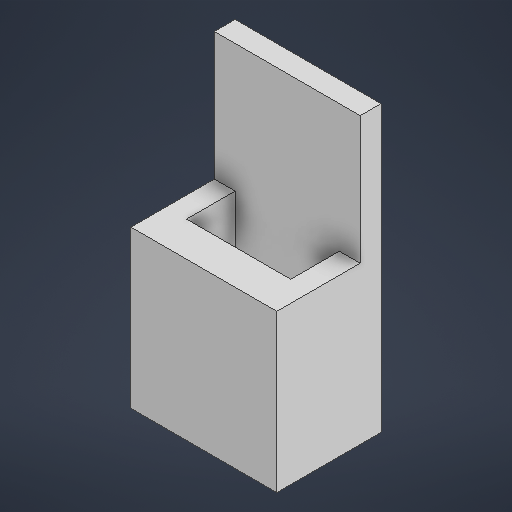
# Autodesk Inventor part: IRsensorhub
Saved by Autodesk Inventor 2026.2 (Build 302298000, 298)
## iProperties
Created: 2026-04-13
Part Number: IRsensorhub
Material: Generic
Document SubType Name: Modeling
Designer: danda
Density: 1 g/cm^3
Appearance: Default
Author: danda
Autodesk Inventor part; units mm, degrees
ref_plane "YZ Plane" through (0, 0, 0) normal (1, 0, 0) x (0, 1, 0)
ref_plane "XZ Plane" through (0, 0, 0) normal (0, 1, 0) x (-1, 0, 0)
ref_plane "XY Plane" through (0, 0, 0) normal (0, 0, 1) x (1, 0, 0)
sketch "Sketch1" plane through (0, 0, 0) normal (0, 0, 1) x (1, 0, 0)
  line L0 (24.1334, 37.8287) -> (39.1334, 37.8287)
  line L1 (39.1334, 37.8287) -> (39.1334, 2.8287)
  line L2 (39.1334, 2.8287) -> (24.1334, 2.8287)
  line L3 (24.1334, 2.8287) -> (24.1334, 37.8287)
  line L4 (42.1334, 40.8287) -> (21.1334, 40.8287)
  line L5 (21.1334, 40.8287) -> (21.1334, -0.1713)
  line L6 (21.1334, -0.1713) -> (42.1334, -0.1713)
  line L7 (42.1334, -0.1713) -> (42.1334, 40.8287)
  line L8 (21.1334, 22.4276) -> (42.1334, 22.4276)
  point P0 (0, 0)
  point P1 (24.1334, 22.4276)
  point P2 (39.1334, 22.4276)
  dimension "d0" = 15
  dimension "d1" = 35
  dimension "d2" = 3
  constraints: 18 end point, 4 parallel, 3 perpendicular, 2 point on line, 1 horizontal, 3 other
  measures "d0" distance of L1.end L2.end
  measures "d1" distance of L0.end L1.end
  measures "d2" distance between parallel lines of L0 L4
extrude "Extrusion1" add sketch "Sketch1" along normal blind 3
extrude "Extrusion2" add sketch "Sketch1" along normal blind 15 contours L3 L2 L1 L8 L7 L6 L5
extrude "Extrusion3" add sketch "Sketch1" along normal blind 15 contours L8 L1 L2 L3
extrude "Extrusion4" cut sketch "Sketch1" along normal blind 10 contours L8 L1 L2 L3
extrude "Extrusion5" add sketch "Sketch1" along normal blind 3 contours L8 L1 L2 L3
sketch "Sketch2" plane through (24.1334, 2.8287, 3) normal (0, 1, 0) x (1, 0, 0)
  line L0 (0, -7) -> (15, -7) projected
  line L1 (3.5, -7) -> (11.5, -7)
  line L2 (11.5, -7) -> (11.5, -2)
  line L3 (11.5, -2) -> (3.5, -2)
  line L4 (3.5, -2) -> (3.5, -7)
  line L5 (0, -7) -> (0, 0) projected
  point P0 (-24.1334, 3)
  dimension "d13" = 8
  dimension "d14" = 5
  dimension "d15" = 3.5
  constraints: 8 end point, 2 parallel, 1 horizontal, 1 perpendicular, 1 point on line
  measures "d13" distance of L3.end L2.end
  measures "d14" distance of L2.end L1.end
  measures "d15" distance between parallel lines of L5 L4
extrude "Extrusion6" cut sketch "Sketch2" against normal blind 3
body "Solid1"
